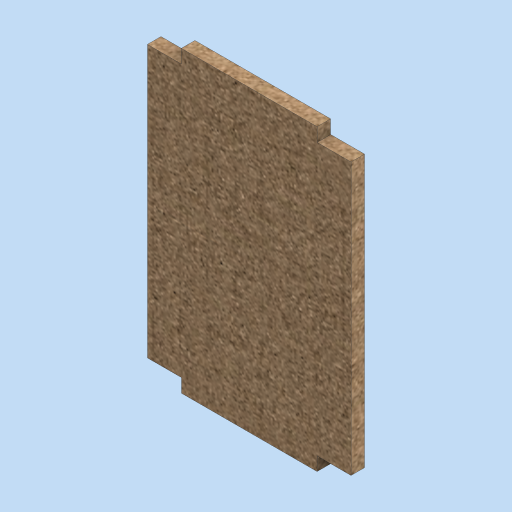
# Autodesk Inventor part: UNION_SOPORTE
Saved by Autodesk Inventor 2024.2 (Build 282272000, 272)
## iProperties
Created: 2024-10-02
Part Number: UNION_SOPORTE
Material: MDF Medium Density Fiberboard
Document SubType Name: Modeling
Designer: jrcer
Density: 0.8 g/cm^3
Appearance: Cardboard - Corrugated
Author: jrcer
Autodesk Inventor part; units mm, degrees
ref_plane "YZ Plane" through (0, 0, 0) normal (1, 0, 0) x (0, 1, 0)
ref_plane "XZ Plane" through (0, 0, 0) normal (0, 1, 0) x (-1, 0, 0)
ref_plane "XY Plane" through (0, 0, 0) normal (0, 0, 1) x (1, 0, 0)
sketch "Sketch1" plane through (0, 0, 0) normal (0, 0, 1) x (1, 0, 0)
  line L0 (-22.5, 30) -> (22.5, 30)
  line L1 (22.5, 30) -> (22.5, -30)
  line L2 (22.5, -30) -> (-22.5, -30)
  line L3 (-22.5, -30) -> (-22.5, 30)
  line L4 (-22.5, 30) -> (22.5, -30) construction
  line L5 (22.5, 30) -> (-22.5, -30) construction
  line L6 (-15, 33) -> (15, 33)
  line L7 (15, 33) -> (15, 30)
  line L8 (15, 30) -> (-15, 30)
  line L9 (-15, 30) -> (-15, 33)
  line L10 (-15, 33) -> (15, 30) construction
  line L11 (15, 33) -> (-15, 30) construction
  line L12 (-15, -30) -> (15, -30)
  line L13 (15, -30) -> (15, -33)
  line L14 (15, -33) -> (-15, -33)
  line L15 (-15, -33) -> (-15, -30)
  line L16 (-15, -30) -> (15, -33) construction
  line L17 (15, -30) -> (-15, -33) construction
  point P0 (0, 0)
  point P1 (0, 31.5)
  point P2 (0, -31.5)
  dimension "d0" = 45
  dimension "d1" = 60
  dimension "d2" = 3
  dimension "d3" = 30
  constraints: 36 end point, 6 midpoint, 6 parallel, 3 horizontal, 3 perpendicular, 2 collinear, 2 equal length, 2 vertical alignment
  measures "d0" distance of L1.end L2.end
  measures "d1" distance of L0.end L1.end
  measures "d2" distance of L6.end L7.end
  measures "d3" distance of L6.start L6.end
extrude "Extrusion1" add sketch "Sketch1" along normal blind 3
body "Solid1"
